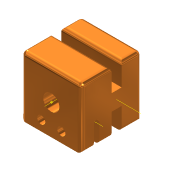
# Autodesk Inventor part: Corredera
Saved by Autodesk Inventor 2021 (Build 250183000, 183)
## iProperties
Created: 2021-07-04
Part Number: Corredera
Material: Iron, Cast
Document SubType Name: Modeling
Designer: Santiago
Density: 7.15 g/cm^3
Appearance: Iron Gray
Mass: 153.696 g
Surface Area: 73.7168 cm^2
Volume: 21.496 cm^3
Author: Santiago
Autodesk Inventor part; units mm, degrees
ref_plane "YZ Plane" through (0, 0, 0) normal (1, 0, 0) x (0, 1, 0)
ref_plane "XZ Plane" through (0, 0, 0) normal (0, 1, 0) x (-1, 0, 0)
ref_plane "XY Plane" through (0, 0, 0) normal (0, 0, 1) x (1, 0, 0)
sketch "Sketch1" plane through (0, 0, 0) normal (0, 0, 1) x (1, 0, 0)
  line L0 (15, -15) -> (-15, -15)
  line L1 (-15, -15) -> (-15, 15)
  line L2 (-15, 15) -> (15, 15)
  line L3 (15, 15) -> (15, -15)
  line L4 (15, -15) -> (-15, 15) construction
  line L5 (-15, -15) -> (15, 15) construction
  point P0 (0, 0)
  dimension "d0" = 30
  dimension "d1" = 30
  constraints: 12 end point, 2 midpoint, 2 parallel, 1 horizontal, 1 perpendicular
  measures "d0" distance of L1.end L2.end
  measures "d1" distance of L0.end L1.end
extrude "Extrusion1" add sketch "Sketch1" against normal blind 20
sketch "Sketch2" plane through (-15, 15, 0) normal (0, 1, 0) x (1, 0, 0)
  line L0 (30, 0) -> (30, 20) projected
  line L1 (0, 5) -> (30, 5)
  line L2 (30, 5) -> (30, 10)
  line L3 (30, 10) -> (0, 10)
  line L4 (0, 10) -> (0, 5)
  line L5 (0, 5) -> (30, 10) construction
  line L6 (30, 5) -> (0, 10) construction
  line L7 (0, 20) -> (30, 20) projected
  point P0 (15, 0)
  point P1 (15, 7.5)
  dimension "d4" = 5
  dimension "d13" = 10
  constraints: 12 end point, 3 midpoint, 2 parallel, 1 horizontal, 1 perpendicular
  measures "d4" distance of L2.end L1.end
  measures "d13" distance between parallel lines of L3 L7
extrude "Extrusion2" cut sketch "Sketch2" against normal blind 11
sketch "Sketch3" plane through (-15, -15, 0) normal (0, -1, 0) x (1, 0, 0)
  line L0 (30, 0) -> (30, -20) projected
  line L1 (0, -5) -> (30, -5)
  line L2 (30, -5) -> (30, -10)
  line L3 (30, -10) -> (0, -10)
  line L4 (0, -10) -> (0, -5)
  line L5 (0, -5) -> (30, -10) construction
  line L6 (30, -5) -> (0, -10) construction
  line L7 (30, -20) -> (0, -20) projected
  point P0 (15, 0)
  point P1 (15, -7.5)
  dimension "d7" = 5
  dimension "d14" = 10
  constraints: 12 end point, 3 midpoint, 2 parallel, 1 horizontal, 1 perpendicular
  measures "d7" distance of L1.end L2.end
  measures "d14" distance between parallel lines of L7 L3
extrude "Extrusion3" cut sketch "Sketch3" against normal blind 11
sketch "Sketch4" plane through (0, 0, 0) normal (0, 0, 1) x (1, 0, 0)
  circle A0 centre (0, 0) radius 4
  dimension "d10" = 8
  constraints: 1 centre point, 1 coincident
  measures "d10" diameter of A0
extrude "Extrusion4" cut sketch "Sketch4" against normal blind 5
sketch "Sketch6" plane through (0, 0, 0) normal (0, 0, 1) x (1, 0, 0)
  line L0 (15, 15) -> (-15, 15) projected
  line L1 (-15, 15) -> (-15, -15) projected
  circle A0 centre (0, 0) radius 4 projected
  line L2 (15, 15) -> (-15, 15) projected
  line L3 (-15, 15) -> (-15, -15) projected
  line L4 (-15, -15) -> (15, -15) projected
  line L5 (15, -15) -> (15, 15) projected
extrude "Extrusion5" add sketch "Sketch6" along normal blind 10
sketch "Sketch7" plane through (15, -15, -20) normal (1, 0, 0) x (0, 0, -1)
  line L0 (-10, 30) -> (-10, 19) projected
  line L1 (-10, 19) -> (-15, 19)
  line L2 (-30, 19) -> (-15, 19) projected
  point P0 (-12.5, 15)
  constraints: 2 end point, 1 point on line
sketch "Sketch8" plane through (15, -15, -20) normal (1, 0, 0) x (0, 0, -1)
  line L0 (-15, 0) -> (-30, 0) projected
  line L1 (-22.5, 0) -> (-22.5, 10) construction
  line L2 (-21.1875, 0) -> (-21.1875, 10)
  line L3 (-23.8125, 10) -> (-23.8125, 0)
  arc A0 (-23.8125, 0) -> (-21.1875, 0) centre (-22.5, 0) ccw
  arc A1 (-21.1875, 10) -> (-23.8125, 10) centre (-22.5, 10) ccw
  point P0 (-20, 15)
  point P1 (-22.5, 5)
  dimension "d17" = 10
  dimension "d18" = 2.625
  constraints: 8 end point, 4 point on circle, 4 tangent, 2 centre point, 2 midpoint, 1 parallel, 1 vertical
  measures "d17" distance of L1.start L1.end
  measures "d18" diameter of A1
extrude "Extrusion6" cut sketch "Sketch8" against normal through all contours L0 L3 A1 L2
sketch "Sketch9" plane through (0, 0, 10) normal (0, 0, 1) x (1, 0, 0)
  line L0 (15, -15) -> (15, -5) projected
  line L1 (15, -15) -> (5, -15)
  line L2 (-15, -15) -> (15, -15) projected
  line L3 (5, -15) -> (5, -10)
  circle A0 centre (5, -10) radius 2
  line L4 (0, 0) -> (0, -15)
  line L5 (-15, -15) -> (-5, -15)
  line L6 (15, -15) -> (-15, -15)
  line L7 (-5, -15) -> (-5, -10)
  circle A1 centre (-5, -10) radius 2
  dimension "d21" = 10
  dimension "d22" = 5
  dimension "d23" = 4
  constraints: 12 end point, 5 symmetric about line, 2 centre point, 2 coincident, 2 point on line, 1 midpoint, 1 perpendicular, 1 other
  measures "d21" distance of L0.start L1.end
  measures "d22" distance of L1.end L3.end
  measures "d23" diameter of A0
extrude "Extrusion7" cut sketch "Sketch9" against normal blind 15
fillet "Fillet1" radius 2 17 edges at (0, 15, 10) (15, 0, 10) (-15, 0, 10) (-15, 15, 2.5) (0, 15, -5) (15, 15, 2.5) (15, -15, -1.9062) (15, -15, 6.9062) (15, 0, -20) (15, 15, -15) (0, 15, -20) (-15, 15, -15) (0, 15, -10) (15, -15, -15) (-15, 0, -20) (-15, -15, -15) (-15, -15, 6.9062)
body "Solid1"
